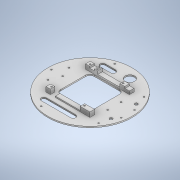
# Autodesk Inventor part: RL_spider_center_top_v3
Saved by Autodesk Inventor 2022 (Build 260153000, 153)
## iProperties
Created: 2021-08-10
Part Number: RL_spider_center_top_v3
Material: Generic
Document SubType Name: Modeling
Designer: Mock
Density: 1 g/cm^3
Appearance: Default
Author: Mock
Autodesk Inventor part; units mm, degrees
ref_plane "YZ Plane" through (0, 0, 0) normal (1, 0, 0) x (0, 1, 0)
ref_plane "XZ Plane" through (0, 0, 0) normal (0, 1, 0) x (-1, 0, 0)
ref_plane "XY Plane" through (0, 0, 0) normal (0, 0, 1) x (1, 0, 0)
sketch "Sketch1" plane through (0, 0, 0) normal (0, 1, 0) x (-1, 0, 0)
  circle A0 centre (0, 0) radius 100
  dimension "d0" = 200
  constraints: 1 centre point, 1 coincident
  measures "d0" diameter of A0
extrude "Extrusion1" add sketch "Sketch1" along normal blind 3
sketch "Sketch2" plane through (0, 3, 0) normal (0, 1, 0) x (1, 0, 0)
  line L0 (0, 0) -> (59.3503, 0)
  circle A0 centre (-92, 0) radius 1.75
  circle A1 centre (-28.4296, -87.4972) radius 1.75
  circle A2 centre (74.4296, -54.0762) radius 1.75
  circle A3 centre (74.4296, 54.0762) radius 1.75
  circle A4 centre (-28.4296, 87.4972) radius 1.75
  dimension "d135" = 3.5
  dimension "d136" = 92
  dimension "d139" = 360
  constraints: 5 centre point, 2 end point, 1 horizontal, 11 other
  measures "d135" diameter of A0
  measures "d136" distance of L0.start A0.centre
extrude "Extrusion2" cut sketch "Sketch2" against normal blind 4
sketch "Sketch3" plane through (0, 3, 0) normal (0, 1, 0) x (1, 0, 0)
  line L0 (-52.25, 52.5) -> (52.25, 52.5)
  line L1 (52.25, 52.5) -> (52.25, 41.5)
  line L2 (52.25, 41.5) -> (-52.25, 41.5)
  line L3 (-52.25, 41.5) -> (-52.25, 52.5)
  line L4 (-52.25, -52.5) -> (52.25, -52.5)
  line L5 (52.25, -52.5) -> (52.25, -41.5)
  line L6 (52.25, -41.5) -> (-52.25, -41.5)
  line L7 (-52.25, -41.5) -> (-52.25, -52.5)
  point P0 (0, 0)
  dimension "d25" = 105
  dimension "d26" = 52.5
  dimension "d27" = 11
  dimension "d28" = 11
  dimension "d29" = 104.5
  dimension "d30" = 104.5
  dimension "d31" = 52.25
  dimension "d32" = 52.25
  constraints: 16 end point, 4 parallel, 2 horizontal, 2 perpendicular
  measures "d25" distance between parallel lines of L0 L4
  measures "d26" distance from line of point (0, 0) L0
  measures "d27" distance of L2.end L0.start
  measures "d28" distance of L6.end L4.start
  measures "d29" distance between parallel lines of L1 L3
  measures "d30" distance of L5.end L6.end
  measures "d31" distance from line of point (0, 0) L7
  measures "d32" distance from line of point (0, 0) L3
extrude "Extrusion3" add sketch "Sketch3" along normal blind 11.2
sketch "Sketch4" plane through (-52.25, 3, 52.5) normal (0, 0, 1) x (1, 0, 0)
  line L0 (0, 11.2) -> (104.5, 11.2) projected
  line L1 (10.25, 11.2) -> (22.25, 11.2)
  line L2 (22.25, 11.2) -> (22.25, 0)
  line L3 (22.25, 0) -> (10.25, 0)
  line L4 (10.25, 0) -> (10.25, 11.2)
  line L5 (22.25, 11.2) -> (81.25, 11.2)
  line L6 (81.25, 11.2) -> (81.25, 2.75)
  line L7 (81.25, 2.75) -> (22.25, 2.75)
  line L8 (22.25, 2.75) -> (22.25, 11.2)
  line L9 (0, 0) -> (0, 11.2) projected
  line L10 (152.25, 0) -> (-47.75, 0) projected
  point P0 (52.25, -3)
  point P1 (22.25, 2.75)
  dimension "d35" = 10.25
  dimension "d36" = 12
  dimension "d37" = 59
  dimension "d38" = 0
  dimension "d39" = 2.75
  constraints: 16 end point, 4 parallel, 2 horizontal, 2 perpendicular, 1 point on line
  measures "d35" distance between parallel lines of L4 L9
  measures "d36" distance between parallel lines of L2 L4
  measures "d37" distance of L6.end L7.end
  measures "d38" distance between parallel lines of L10 L3
  measures "d39" distance between parallel lines of L10 L7
extrude "Extrusion4" cut sketch "Sketch4" against normal blind 11 contours L0 L2 L3 L4 | L0 L6 L7 L2
sketch "Sketch5" plane through (-52.25, 3, -41.5) normal (0, 0, 1) x (1, 0, 0)
  line L0 (0, 11.2) -> (104.5, 11.2) projected
  line L1 (10.15, 11.2) -> (20.95, 11.2)
  line L2 (20.95, 11.2) -> (20.95, 7.25)
  line L3 (20.95, 7.25) -> (10.15, 7.25)
  line L4 (10.15, 7.25) -> (10.15, 11.2)
  line L5 (29.2, 11.2) -> (81.85, 11.2)
  line L6 (81.85, 11.2) -> (81.85, 4)
  line L7 (81.85, 4) -> (29.2, 4)
  line L8 (29.2, 4) -> (29.2, 11.2)
  line L9 (93.5, 11.2) -> (104.5, 11.2)
  line L10 (104.5, 11.2) -> (104.5, 7.3)
  line L11 (104.5, 7.3) -> (93.5, 7.3)
  line L12 (93.5, 7.3) -> (93.5, 11.2)
  line L13 (0, 0) -> (0, 11.2) projected
  line L14 (104.5, 0) -> (0, 0) projected
  line L15 (104.5, 0) -> (104.5, 11.2) projected
  point P0 (52.25, -3)
  dimension "d42" = 10.15
  dimension "d43" = 10.8
  dimension "d44" = 8.25
  dimension "d45" = 52.65
  dimension "d46" = 11.65
  dimension "d47" = 7.3
  dimension "d48" = 4
  dimension "d49" = 7.25
  dimension "d51" = 11
  constraints: 24 end point, 6 parallel, 3 horizontal, 3 perpendicular, 3 point on line
  measures "d42" distance between parallel lines of L4 L13
  measures "d43" distance of L2.end L3.end
  measures "d44" distance between parallel lines of L8 L2
  measures "d45" distance of L6.end L7.end
  measures "d46" distance between parallel lines of L12 L6
  measures "d47" distance between parallel lines of L14 L11
  measures "d48" distance between parallel lines of L14 L7
  measures "d49" distance between parallel lines of L14 L3
  measures "d51" distance of L10.end L11.end
extrude "Extrusion5" cut sketch "Sketch5" against normal blind 11 contours L0 L2 L3 L4 | L0 L6 L7 L8 | L11 L12 L0 L10
sketch "Sketch6" plane through (0, 3, 0) normal (0, 1, 0) x (1, 0, 0)
  circle A0 centre (80, 30) radius 3.5
  circle A1 centre (80, -30) radius 3.5
  line L0 (-30, 40) -> (30, 40)
  line L1 (40, 30) -> (40, -30)
  line L2 (30, -40) -> (-30, -40)
  line L3 (-40, -30) -> (-40, 30)
  line L4 (-31.3, 41.5) -> (-42.1, 41.5) projected
  line L5 (-30, -41.5) -> (29, -41.5) projected
  line L6 (-52.25, -41.5) -> (-52.25, -52.5) projected
  line L7 (52.25, -52.5) -> (52.25, -41.5) projected
  arc A2 (-30, 40) -> (-40, 30) centre (-30, 30) ccw
  arc A3 (40, 30) -> (30, 40) centre (30, 30) ccw
  arc A4 (30, -40) -> (40, -30) centre (30, -30) ccw
  arc A5 (-40, -30) -> (-30, -40) centre (-30, -30) ccw
  point P0 (0, 0)
  dimension "d54" = 30
  dimension "d55" = 30
  dimension "d56" = 80
  dimension "d57" = 80
  dimension "d58" = 7
  dimension "d59" = 7
  dimension "d127" = 80
  dimension "d128" = 40
  dimension "d129" = 80
  dimension "d130" = 40
  dimension "d131" = 10
  constraints: 8 end point, 8 point on circle, 8 tangent, 6 centre point, 3 equal radius, 2 parallel, 1 horizontal, 1 perpendicular
  measures "d54" vertical distance of point (0, 0) A0.centre
  measures "d55" vertical distance of point (0, 0) A1.centre
  measures "d56" horizontal distance of A0.centre point (0, 0)
  measures "d57" horizontal distance of A1.centre point (0, 0)
  measures "d58" diameter of A1
  measures "d59" diameter of A0
  measures "d127" distance between parallel lines of L1 L3
  measures "d128" distance from line of point (0, 0) L3
  measures "d129" distance between parallel lines of L2 L0
  measures "d130" distance from line of point (0, 0) L2
  measures "d131" radius of A2
extrude "Extrusion6" cut sketch "Sketch6" against normal blind 11
sketch "Sketch7" plane through (0, 14.2, 0) normal (0, 1, 0) x (1, 0, 0)
  line L0 (-52.25, 52.5) -> (52.25, 52.5) projected
  line L1 (-29.175, 52.5) -> (-25.175, 52.5)
  line L2 (-25.175, 52.5) -> (-25.175, 43.5)
  line L3 (-25.175, 43.5) -> (-29.175, 43.5)
  line L4 (-29.175, 43.5) -> (-29.175, 52.5)
  line L5 (-31.3, 52.5) -> (-31.3, 41.5) projected
  line L6 (-31.3, 41.5) -> (-23.05, 41.5) projected
  point P0 (0, 0)
  dimension "d65" = 4
  dimension "d66" = 2.125
  dimension "d67" = 2
  constraints: 8 end point, 2 parallel, 1 horizontal, 1 perpendicular, 1 point on line
  measures "d65" distance between parallel lines of L2 L4
  measures "d66" distance between parallel lines of L4 L5
  measures "d67" distance between parallel lines of L6 L3
extrude "Extrusion7" cut sketch "Sketch7" against normal blind 2
sketch "Sketch8" plane through (0, 14.2, 0) normal (0, 1, 0) x (1, 0, 0)
  circle A0 centre (32.75, -46) radius 1.75
  line L0 (52.25, -52.5) -> (52.25, -41.5) projected
  line L1 (29, -52.5) -> (52.25, -52.5) projected
  circle A1 centre (-45.75, -46) radius 1.75
  circle A2 centre (-45.75, 46) radius 1.75
  circle A3 centre (32.75, 46) radius 1.75
  line L2 (52.25, 52.5) -> (52.25, 41.5) projected
  line L3 (41.25, 52.5) -> (29.6, 52.5) projected
  line L4 (-42.1, 52.5) -> (-52.25, 52.5) projected
  line L5 (-52.25, -41.5) -> (-52.25, -52.5) projected
  line L6 (-52.25, -52.5) -> (-42, -52.5) projected
  line L7 (-52.25, 52.5) -> (-52.25, 41.5) projected
  point P0 (0, 0)
  dimension "d70" = 19.5
  dimension "d71" = 6.5
  dimension "d72" = 3.5
  dimension "d73" = 19.5
  dimension "d74" = 6.5
  dimension "d75" = 3.5
  dimension "d76" = 6.5
  dimension "d77" = 6.5
  dimension "d78" = 6.5
  dimension "d79" = 6.5
  dimension "d80" = 3.5
  dimension "d81" = 3.5
  constraints: 4 centre point
  measures "d70" distance from line of L0 A0.centre
  measures "d71" distance from line of L1 A0.centre
  measures "d72" diameter of A0
  measures "d73" distance from line of L2 A3.centre
  measures "d74" distance from line of L3 A3.centre
  measures "d75" diameter of A3
  measures "d76" distance from line of L4 A2.centre
  measures "d77" distance from line of A1.centre L5
  measures "d78" distance from line of A1.centre L6
  measures "d79" distance from line of A2.centre L7
  measures "d80" diameter of A2
  measures "d81" diameter of A1
extrude "Extrusion8" cut sketch "Sketch8" against normal blind 18.2
sketch "Sketch9" plane through (0, 3, 0) normal (0, 1, 0) x (1, 0, 0)
  arc A0 (30, -76) -> (30, -64) centre (30, -70) ccw
  arc A1 (-40, -64) -> (-40, -76) centre (-40, -70) ccw
  line L0 (-40, -64) -> (30, -64)
  line L1 (-40, -76) -> (30, -76)
  point P0 (0, 0)
  dimension "d84" = 12
  dimension "d86" = 70
  dimension "d87" = 40
  dimension "d88" = 70
  dimension "d89" = 70
  dimension "d90" = 12
  constraints: 4 end point, 4 point on circle, 2 centre point, 1 parallel, 1 tangent
  measures "d84" diameter of A0
  measures "d86" vertical distance of A1.centre point (0, 0)
  measures "d87" horizontal distance of point (0, 0) A1.centre
  measures "d88" distance of A0.centre A1.centre
  measures "d89" vertical distance of A0.centre point (0, 0)
  measures "d90" diameter of A1
extrude "Extrusion9" cut sketch "Sketch9" against normal blind 4
sketch "Sketch10" plane through (0, 3, 0) normal (0, 1, 0) x (1, 0, 0)
  circle A0 centre (-75, 25) radius 1.75
  circle A1 centre (-75, -25) radius 1.75
  circle A2 centre (-65, 0) radius 1.75
  point P0 (0, 0)
  dimension "d94" = 50
  dimension "d95" = 75
  dimension "d96" = 3.5
  dimension "d97" = 3.5
  dimension "d120" = 25
  dimension "d121" = 75
  dimension "d132" = 3.5
  dimension "d133" = 65
  dimension "d134" = 25
  constraints: 3 centre point
  measures "d94" distance of A1.centre A0.centre
  measures "d95" horizontal distance of point (0, 0) A1.centre
  measures "d96" diameter of A1
  measures "d97" diameter of A0
  measures "d120" vertical distance of point (0, 0) A1.centre
  measures "d121" horizontal distance of point (0, 0) A0.centre
  measures "d132" diameter of A2
  measures "d133" distance of A2.centre point (0, 0)
  measures "d134" vertical distance of A2.centre A0.centre
extrude "Extrusion10" cut sketch "Sketch10" against normal blind 11
sketch "Sketch13" plane through (0, 3, 0) normal (0, 1, 0) x (1, 0, 0)
  arc A0 (-15, 64) -> (-15, 76) centre (-15, 70) ccw
  circle A1 centre (0, 0) radius 100 projected
  line L0 (52.25, 52.5) -> (52.25, 41.5) projected
  circle A2 centre (20, 75) radius 11.25
  arc A3 (-40, 76) -> (-40, 64) centre (-40, 70) ccw
  line L1 (-40, 64) -> (-15, 64)
  line L2 (-40, 76) -> (-15, 76)
  dimension "d107" = 12
  dimension "d111" = 22.5
  dimension "d112" = 20
  dimension "d113" = 15
  dimension "d114" = 70
  dimension "d115" = 75
  dimension "d160" = 25
  dimension "d161" = 12
  constraints: 4 end point, 4 point on circle, 4 tangent, 3 centre point
  measures "d107" diameter of A0
  measures "d111" diameter of A2
  measures "d112" horizontal distance of A2.centre point (0, 0)
  measures "d113" horizontal distance of A0.centre point (0, 0)
  measures "d114" vertical distance of A0.centre point (0, 0)
  measures "d115" vertical distance of A2.centre point (0, 0)
  measures "d160" distance of A0.centre A3.centre
  measures "d161" diameter of A3
extrude "Extrusion12" cut sketch "Sketch13" against normal blind 11.2 contours L1 A3 L2 A0 | A2
sketch "Sketch16" plane through (0, 3, 0) normal (0, 1, 0) x (1, 0, 0)
  line L0 (54, 20) -> (94, 20)
  line L1 (94, 20) -> (94, -20)
  line L2 (94, -20) -> (54, -20)
  line L3 (54, -20) -> (54, 20)
  circle A0 centre (0, 0) radius 100 projected
  circle A1 centre (0, 0) radius 97
  line L4 (94, 20) -> (94.9158, 20)
  circle A2 centre (58, 16) radius 1.75
  circle A3 centre (90, 16) radius 1.75
  circle A4 centre (58, -16) radius 1.75
  circle A5 centre (90, -16) radius 1.75
  line L5 (-30, 40) -> (30, 40) projected
  dimension "d141" = 40
  dimension "d142" = 40
  dimension "d143" = 20
  dimension "d144" = 3
  dimension "d146" = 4
  dimension "d147" = 4
  dimension "d148" = 4
  dimension "d149" = 4
  dimension "d150" = 4
  dimension "d151" = 4
  dimension "d152" = 4
  dimension "d153" = 4
  dimension "d154" = 3.5
  dimension "d155" = 3.5
  dimension "d156" = 3.5
  dimension "d157" = 3.5
  dimension "d162" = 54
  constraints: 10 end point, 4 centre point, 3 parallel, 2 horizontal, 1 coincident, 1 perpendicular, 3 other
  measures "d141" distance of L0.start L0.end
  measures "d142" distance of L0.end L1.end
  measures "d143" distance from line of point (0, 0) L0
  measures "d146" distance from line of L0 A2.centre
  measures "d147" distance from line of A2.centre L3
  measures "d148" distance from line of L0 A3.centre
  measures "d149" distance from line of L1 A3.centre
  measures "d150" distance from line of L2 A4.centre
  measures "d151" distance from line of L3 A4.centre
  measures "d152" distance from line of L2 A5.centre
  measures "d153" distance from line of L1 A5.centre
  measures "d154" diameter of A5
  measures "d155" diameter of A4
  measures "d156" diameter of A2
  measures "d157" diameter of A3
  measures "d162" distance from line of L3 A0.centre
extrude "Extrusion14" cut sketch "Sketch16" against normal blind 10 contours A2 | A3 | A4 | A5
equation "\"d26\" = 0.5 * d25"
equation "\"d31\" = 0.5 * d30"
equation "\"d32\" = 0.5 * d29"
equation "\"d128\" = 0.5 * d127"
equation "\"d130\" = 0.5 * d129"
body "Solid1"
